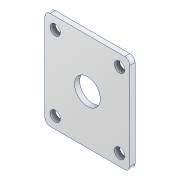
# Autodesk Inventor part: castor_top
Saved by Autodesk Inventor 2020 (Build 240168000, 168)
## iProperties
Created: 2020-09-08
Part Number: castor_top
Material: 알루미늄 6061
Document SubType Name: Modeling
Designer: 이호석
Mass: 6.05751 g
Surface Area: 26.8402 cm^2
Volume: 2.24352 cm^3
Density: 2.7 g/cm^3
Appearance: 알루미늄 - 평지
Author: 이호석
Autodesk Inventor part; units mm, degrees
ref_plane "YZ Plane" through (0, 0, 0) normal (1, 0, 0) x (0, 1, 0)
ref_plane "XZ Plane" through (0, 0, 0) normal (0, 1, 0) x (-1, 0, 0)
ref_plane "XY Plane" through (0, 0, 0) normal (0, 0, 1) x (1, 0, 0)
sketch "스케치1" plane through (0, 0, 0) normal (0, 0, 1) x (1, 0, 0)
  line L0 (16.5, -19) -> (-16.5, -19)
  line L1 (-16.5, -19) -> (-16.5, 19)
  line L2 (-16.5, 19) -> (16.5, 19)
  line L3 (16.5, 19) -> (16.5, -19)
  line L4 (16.5, -19) -> (-16.5, 19) construction
  line L5 (-16.5, -19) -> (16.5, 19) construction
  line L6 (12.5, -14.5) -> (-12.5, -14.5)
  line L7 (-12.5, -14.5) -> (-12.5, 14.5)
  line L8 (-12.5, 14.5) -> (12.5, 14.5)
  line L9 (12.5, 14.5) -> (12.5, -14.5)
  line L10 (12.5, -14.5) -> (-12.5, 14.5) construction
  line L11 (-12.5, -14.5) -> (12.5, 14.5) construction
  circle A0 centre (-12.5, 14.5) radius 2
  circle A1 centre (12.5, 14.5) radius 2
  circle A2 centre (12.5, -14.5) radius 2
  circle A3 centre (-12.5, -14.5) radius 2
  point P0 (0, 0)
  dimension "d14" = 33
  dimension "d15" = 38
  dimension "d16" = 25
  dimension "d17" = 29
  dimension "d18" = 4
  dimension "d19" = 4
  dimension "d20" = 4
  dimension "d21" = 4
  constraints: 24 end point, 4 centre point, 4 coincident, 4 midpoint, 4 parallel, 2 horizontal, 2 perpendicular
  measures "d14" distance of L1.end L2.end
  measures "d15" distance of L0.end L1.end
  measures "d16" distance of L7.end L8.end
  measures "d17" distance of L6.end L7.end
  measures "d18" diameter of A0
  measures "d19" diameter of A1
  measures "d20" diameter of A2
  measures "d21" diameter of A3
extrude "돌출1" add sketch "스케치1" along normal blind 2 contours L0 L1 L2 L3 | A3 L7 A0 L8 A1 L9 A2 L6
fillet "모깎기1" radius 2 4 edges at (-16.5, 19, 1) (16.5, 19, 1) (16.5, -19, 1) (-16.5, -19, 1)
sketch "스케치2" plane through (0, 0, 2) normal (0, 0, 1) x (1, 0, 0)
  circle A0 centre (0, 0) radius 5
  dimension "d11" = 10
  constraints: 1 centre point, 1 coincident
  measures "d11" diameter of A0
extrude "돌출2" cut sketch "스케치2" against normal through all
